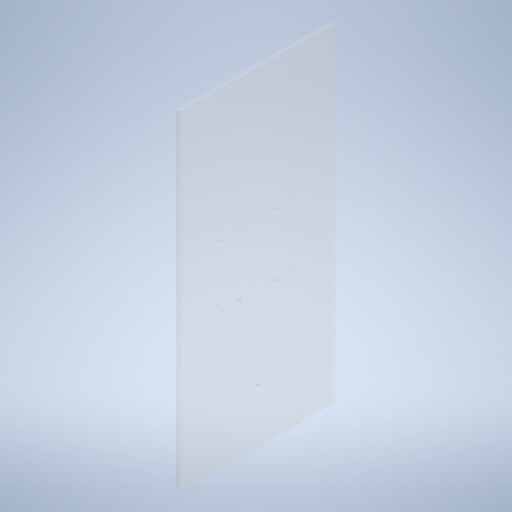
# Autodesk Inventor part: 발판
Saved by Autodesk Inventor 2024 (Build 280153000, 153)
## iProperties
Created: 2024-04-13
Part Number: 발판
Material: PMMA 플라스틱
Document SubType Name: Modeling
Designer: kkamin5
Density: 1.188 g/cm^3
Appearance: 폴리카보네이트 - 선명
Mass: 119.347 g
Surface Area: 698.631 cm^2
Volume: 100.461 cm^3
Author: kkamin5
Autodesk Inventor part; units mm, degrees
ref_plane "YZ Plane" through (0, 0, 0) normal (1, 0, 0) x (0, 1, 0)
ref_plane "XZ Plane" through (0, 0, 0) normal (0, 1, 0) x (-1, 0, 0)
ref_plane "XY Plane" through (0, 0, 0) normal (0, 0, 1) x (1, 0, 0)
sketch "스케치1" plane through (0, 0, 0) normal (1, 0, 0) x (0, 1, 0)
  line L0 (-160, 75) -> (160, 75)
  line L1 (160, 75) -> (160, -75)
  line L2 (160, -75) -> (-160, -75)
  line L3 (-160, -75) -> (-160, 75)
  line L4 (-160, 75) -> (160, -75) construction
  line L5 (160, 75) -> (-160, -75) construction
  point P0 (0, 0)
  dimension "d0" = 320
  dimension "d1" = 150
  constraints: 12 end point, 2 midpoint, 2 parallel, 1 horizontal, 1 perpendicular
  measures "d0" distance of L1.end L2.end
  measures "d1" distance of L0.end L1.end
extrude "돌출1" add sketch "스케치1" along normal mid plane 3
sketch "스케치2" plane through (-1.5, 0, 0) normal (-1, 0, 0) x (0, 0, 1)
  line L0 (-75, -160) -> (75, -160) projected
  point P0 (0, 0)
  point P1 (0, -110)
  point P2 (-17.5, 30)
  point P3 (-35, 30)
  point P4 (-35, -30)
  point P5 (-17.5, -30)
  point P6 (17.5, 30)
  point P7 (35, 30)
  point P8 (35, -30)
  point P9 (17.5, -30)
  dimension "d11" = 50
  dimension "d19" = 110
  dimension "d20" = 30
  dimension "d21" = 30
  dimension "d22" = 30
  dimension "d23" = 30
  dimension "d24" = 30
  dimension "d25" = 30
  dimension "d26" = 30
  dimension "d27" = 30
  dimension "d28" = 35
  dimension "d29" = 35
  dimension "d30" = 35
  dimension "d31" = 35
  dimension "d32" = 17.5
  dimension "d33" = 17.5
  dimension "d34" = 17.5
  dimension "d35" = 17.5
  measures "d11" distance from line of point (0, -110) L0
  measures "d19" distance of point (0, 0) point (0, -110)
  measures "d20" vertical distance of point (0, 0) point (-17.5, 30)
  measures "d21" vertical distance of point (0, 0) point (-17.5, -30)
  measures "d22" vertical distance of point (0, 0) point (-35, -30)
  measures "d23" vertical distance of point (0, 0) point (-35, 30)
  measures "d24" vertical distance of point (0, 0) point (17.5, -30)
  measures "d25" vertical distance of point (0, 0) point (35, -30)
  measures "d26" vertical distance of point (0, 0) point (35, 30)
  measures "d27" vertical distance of point (0, 0) point (17.5, 30)
  measures "d28" horizontal distance of point (0, 0) point (-35, 30)
  measures "d29" horizontal distance of point (-35, -30) point (0, 0)
  measures "d30" horizontal distance of point (35, -30) point (0, 0)
  measures "d31" horizontal distance of point (0, 0) point (35, 30)
  measures "d32" horizontal distance of point (-17.5, -30) point (0, 0)
  measures "d33" horizontal distance of point (0, 0) point (-17.5, 30)
  measures "d34" horizontal distance of point (0, 0) point (17.5, 30)
  measures "d35" horizontal distance of point (0, 0) point (17.5, -30)
hole "구멍1" at (-1.5, -110, 0) at (-1.5, 30, -17.5) at (-1.5, 30, -35) at (-1.5, -30, -35) at (-1.5, -30, -17.5) at (-1.5, -30, 17.5) at (-1.5, 30, 17.5) at (-1.5, 30, 35) at (-1.5, -30, 35) direction (1, 0, 0) diameter 4 end through all
equation "\"d32\" = 0.5 * d29"
equation "\"d33\" = 0.5 * d28"
equation "\"d34\" = 0.5 * d31"
equation "\"d35\" = d34"
